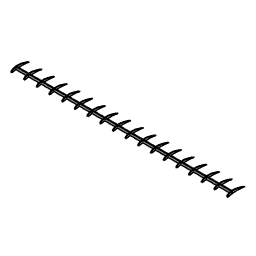
Boeing wing v1 (Autodesk Fusion 360 design; units mm, degrees)
Autodesk Fusion 360 part; units mm, degrees
note: some values were not read from the file. Set by a fixed rule: which sketch regions a step uses.
sketch "E423_1.0" plane through (0, 0, 0) normal (1, 0, 0) x (0, 0, -1)
  spline S0 degree 5 poles (0, 100) (-0.0021, 100.0005) (-0.0141, 99.9805) (-0.0559, 99.8873) (-0.1498, 99.6703) (-0.2899, 99.3695) (-0.4368, 99.0842) (-0.5908, 98.8088) (-0.7588, 98.5154) (-0.9439, 98.1889) (-1.1433, 97.8316) (-1.352, 97.4534) (-1.5644, 97.0669) (-1.7766, 96.6789) (-1.9869, 96.2896) (-2.1952, 95.8959) (-2.4017, 95.4928) (-2.607, 95.0764) (-2.8112, 94.6453) (-3.0137, 94.2001) (-3.2143, 93.7424) (-3.4125, 93.2744) (-3.6081, 92.7977) (-3.8013, 92.3132) (-3.9926, 91.8213) (-4.1824, 91.3216) (-4.3714, 90.8138) (-4.5601, 90.2978) (-4.7489, 89.7736) (-4.9377, 89.2414) (-5.1267, 88.7019) (-5.3157, 88.1556) (-5.5046, 87.6032) (-5.6933, 87.0452) (-5.8819, 86.4818) (-6.0702, 85.9134) (-6.2583, 85.34) (-6.4462, 84.7617) (-6.634, 84.1786) (-6.8217, 83.5907) (-7.0093, 82.9982) (-7.1967, 82.4013) (-7.3839, 81.8002) (-7.5709, 81.1951) (-7.7576, 80.5861) (-7.9439, 79.9736) (-8.1298, 79.3577) (-8.3152, 78.7385) (-8.5002, 78.1162) (-8.6845, 77.4909) (-8.8682, 76.8626) (-9.0513, 76.2315) (-9.2336, 75.5977) (-9.4152, 74.9612) (-9.596, 74.3223) (-9.7758, 73.681) (-9.9548, 73.0374) (-10.1328, 72.3916) (-10.3098, 71.7438) (-10.4856, 71.0941) (-10.6604, 70.4425) (-10.8339, 69.7892) (-11.0061, 69.1343) (-11.177, 68.4777) (-11.3465, 67.8197) (-11.5145, 67.1603) (-11.6809, 66.4996) (-11.8456, 65.8377) (-12.0086, 65.1746) (-12.1697, 64.5105) (-12.3289, 63.8455) (-12.4861, 63.1796) (-12.6411, 62.513) (-12.794, 61.8456) (-12.9446, 61.1777) (-13.0928, 60.5092) (-13.2386, 59.8402) (-13.3819, 59.1708) (-13.5226, 58.5011) (-13.6606, 57.8311) (-13.7958, 57.1609) (-13.9281, 56.4907) (-14.0573, 55.8205) (-14.1834, 55.1503) (-14.3061, 54.4803) (-14.4254, 53.8106) (-14.5409, 53.1412) (-14.6526, 52.4721) (-14.7601, 51.8034) (-14.8634, 51.1351) (-14.9621, 50.4673) (-15.0562, 49.7999) (-15.1453, 49.133) (-15.2294, 48.4665) (-15.3085, 47.8005) (-15.3823, 47.135) (-15.4509, 46.4699) (-15.5142, 45.8053) (-15.5722, 45.1412) (-15.6248, 44.4777) (-15.6722, 43.8147) (-15.7141, 43.1524) (-15.7507, 42.4907) (-15.7819, 41.8299) (-15.8077, 41.1698) (-15.8281, 40.5107) (-15.8431, 39.8526) (-15.8526, 39.1955) (-15.8567, 38.5395) (-15.8553, 37.8847) (-15.8485, 37.2311) (-15.8364, 36.5788) (-15.8188, 35.9278) (-15.7958, 35.2782) (-15.7674, 34.6301) (-15.7337, 33.9835) (-15.6946, 33.3387) (-15.6501, 32.6956) (-15.6003, 32.0543) (-15.5451, 31.4149) (-15.4846, 30.7776) (-15.4187, 30.1423) (-15.3476, 29.5091) (-15.2711, 28.8782) (-15.1893, 28.2495) (-15.1023, 27.6231) (-15.0101, 26.9992) (-14.9128, 26.3778) (-14.8103, 25.759) (-14.7029, 25.143) (-14.5905, 24.5298) (-14.4731, 23.9196) (-14.351, 23.3125) (-14.224, 22.7085) (-14.0923, 22.1078) (-13.9558, 21.5106) (-13.8146, 20.9168) (-13.6687, 20.3268) (-13.5181, 19.7405) (-13.3628, 19.1581) (-13.2028, 18.5797) (-13.0381, 18.0056) (-12.8687, 17.4357) (-12.6946, 16.8704) (-12.5159, 16.3097) (-12.3324, 15.7538) (-12.1444, 15.2029) (-11.9517, 14.6571) (-11.7543, 14.1166) (-11.5524, 13.5816) (-11.3459, 13.0522) (-11.1347, 12.5286) (-10.9189, 12.0109) (-10.6985, 11.4994) (-10.4735, 10.9943) (-10.2439, 10.4956) (-10.0096, 10.0037) (-9.7708, 9.5188) (-9.5273, 9.0412) (-9.2793, 8.571) (-9.0267, 8.1087) (-8.7697, 7.6544) (-8.5081, 7.2084) (-8.242, 6.771) (-7.9714, 6.3424) (-7.6963, 5.9229) (-7.4168, 5.513) (-7.1328, 5.1129) (-6.8444, 4.7231) (-6.5517, 4.3441) (-6.2547, 3.9762) (-5.9535, 3.62) (-5.6482, 3.2758) (-5.339, 2.9439) (-5.026, 2.625) (-4.7093, 2.3195) (-4.3891, 2.0282) (-4.0654, 1.7521) (-3.7383, 1.4922) (-3.4081, 1.2494) (-3.0753, 1.0245) (-2.7405, 0.8182) (-2.4045, 0.631) (-2.068, 0.4639) (-1.731, 0.3184) (-1.3931, 0.1973) (-1.0564, 0.103) (-0.7276, 0.0376) (-0.4228, 0.002) (-0.1632, -0.0059) (0.0354, 0.0078) (0.1775, 0.0302) (0.2843, 0.0476) (0.4091, 0.0826) (0.5351, 0.1305) (0.5811, 0.1515) (0.6519, 0.1886) (0.7136, 0.2323) (0.761, 0.2722) (0.8195, 0.3458) (0.8528, 0.3794) (0.9164, 0.4784) (0.9928, 0.6103) (1.0394, 0.7024) (1.101, 0.8594) (1.1715, 1.0486) (1.2233, 1.1907) (1.263, 1.3363) (1.3115, 1.5827) (1.3717, 1.9493) (1.4357, 2.4065) (1.4906, 2.9015) (1.5254, 3.3859) (1.537, 3.8426) (1.5274, 4.2759) (1.5021, 4.7023) (1.4672, 5.142) (1.427, 5.6084) (1.3827, 6.1039) (1.334, 6.6247) (1.2793, 7.163) (1.2169, 7.7103) (1.1456, 8.2603) (1.0652, 8.8106) (0.9763, 9.362) (0.8798, 9.9165) (0.7769, 10.4775) (0.6688, 11.0479) (0.5564, 11.6293) (0.44, 12.2223) (0.3199, 12.8262) (0.1963, 13.44) (0.0692, 14.0622) (-0.0614, 14.6916) (-0.1951, 15.3272) (-0.3316, 15.9686) (-0.4704, 16.6157) (-0.6109, 17.2689) (-0.7524, 17.9285) (-0.8944, 18.595) (-1.0364, 19.2686) (-1.178, 19.9494) (-1.3187, 20.6373) (-1.4584, 21.3321) (-1.5969, 22.0334) (-1.734, 22.7408) (-1.8696, 23.4538) (-2.0037, 24.1721) (-2.1361, 24.8953) (-2.2667, 25.6233) (-2.3954, 26.356) (-2.5219, 27.0932) (-2.6461, 27.8348) (-2.768, 28.581) (-2.8871, 29.3315) (-3.0035, 30.0864) (-3.1169, 30.8455) (-3.2271, 31.6086) (-3.334, 32.3756) (-3.4373, 33.1464) (-3.537, 33.9205) (-3.6328, 34.6979) (-3.7247, 35.4783) (-3.8125, 36.2614) (-3.8962, 37.047) (-3.9757, 37.8349) (-4.0509, 38.6249) (-4.1218, 39.4168) (-4.1886, 40.2103) (-4.251, 41.0052) (-4.3093, 41.8014) (-4.3636, 42.5986) (-4.4138, 43.3968) (-4.4601, 44.1956) (-4.5027, 44.9951) (-4.5417, 45.7949) (-4.5772, 46.595) (-4.6094, 47.3953) (-4.6383, 48.1955) (-4.6641, 48.9956) (-4.6868, 49.7956) (-4.7066, 50.5952) (-4.7235, 51.3944) (-4.7375, 52.1931) (-4.7486, 52.9912) (-4.757, 53.7886) (-4.7625, 54.5852) (-4.7653, 55.381) (-4.7653, 56.1759) (-4.7626, 56.9698) (-4.7572, 57.7626) (-4.749, 58.5542) (-4.7381, 59.3445) (-4.7246, 60.1334) (-4.7083, 60.9208) (-4.6893, 61.7067) (-4.6675, 62.4907) (-4.643, 63.273) (-4.6157, 64.0532) (-4.5856, 64.8313) (-4.5526, 65.6072) (-4.5169, 66.3806) (-4.4783, 67.1516) (-4.4368, 67.9198) (-4.3925, 68.6853) (-4.3454, 69.4479) (-4.2956, 70.2074) (-4.2429, 70.9637) (-4.1876, 71.7167) (-4.1296, 72.4662) (-4.0691, 73.2121) (-4.0062, 73.9541) (-3.9408, 74.692) (-3.8733, 75.4257) (-3.8036, 76.155) (-3.7319, 76.8796) (-3.6583, 77.5994) (-3.5828, 78.3144) (-3.5056, 79.0244) (-3.4265, 79.7294) (-3.3458, 80.4295) (-3.2633, 81.1245) (-3.1792, 81.8143) (-3.0936, 82.4989) (-3.0064, 83.178) (-2.9178, 83.8512) (-2.828, 84.5182) (-2.7372, 85.1783) (-2.6455, 85.8312) (-2.5531, 86.4765) (-2.46, 87.1139) (-2.3662, 87.7434) (-2.2717, 88.3655) (-2.1762, 88.9803) (-2.0795, 89.5885) (-1.9817, 90.1902) (-1.8828, 90.7851) (-1.783, 91.3726) (-1.683, 91.9512) (-1.5834, 92.519) (-1.485, 93.0737) (-1.3883, 93.6141) (-1.2935, 94.1394) (-1.2, 94.6507) (-1.1064, 95.1508) (-1.0112, 95.6433) (-0.9131, 96.1306) (-0.8119, 96.6128) (-0.709, 97.0855) (-0.6082, 97.5386) (-0.5141, 97.9598) (-0.4296, 98.3413) (-0.3539, 98.6832) (-0.2795, 99.003) (-0.1955, 99.3254) (-0.1004, 99.6525) (-0.0298, 99.88) (-0.0015, 99.9772) (0.0021, 99.9995) (0, 100) knots 0 0 0 0 0 0 0.0028169 0.0056338 0.0084507 0.01126761 0.01408451 0.01690141 0.01971831 0.02253521 0.02535211 0.02816901 0.03098592 0.03380282 0.03661972 0.03943662 0.04225352 0.04507042 0.04788732 0.05070423 0.05352113 0.05633803 0.05915493 0.06197183 0.06478873 0.06760563 0.07042254 0.07323944 0.07605634 0.07887324 0.08169014 0.08450704 0.08732394 0.09014085 0.09295775 0.09577465 0.09859155 0.10140845 0.10422535 0.10704225 0.10985915 0.11267606 0.11549296 0.11830986 0.12112676 0.12394366 0.12676056 0.12957746 0.13239437 0.13521127 0.13802817 0.14084507 0.14366197 0.14647887 0.14929577 0.15211268 0.15492958 0.15774648 0.16056338 0.16338028 0.16619718 0.16901408 0.17183099 0.17464789 0.17746479 0.18028169 0.18309859 0.18591549 0.18873239 0.1915493 0.1943662 0.1971831 0.2 0.2028169 0.2056338 0.2084507 0.21126761 0.21408451 0.21690141 0.21971831 0.22253521 0.22535211 0.22816901 0.23098592 0.23380282 0.23661972 0.23943662 0.24225352 0.24507042 0.24788732 0.25070423 0.25352113 0.25633803 0.25915493 0.26197183 0.26478873 0.26760563 0.27042254 0.27323944 0.27605634 0.27887324 0.28169014 0.28450704 0.28732394 0.29014085 0.29295775 0.29577465 0.29859155 0.30140845 0.30422535 0.30704225 0.30985915 0.31267606 0.31549296 0.31830986 0.32112676 0.32394366 0.32676056 0.32957746 0.33239437 0.33521127 0.33802817 0.34084507 0.34366197 0.34647887 0.34929577 0.35211268 0.35492958 0.35774648 0.36056338 0.36338028 0.36619718 0.36901408 0.37183099 0.37464789 0.37746479 0.38028169 0.38309859 0.38591549 0.38873239 0.3915493 0.3943662 0.3971831 0.4 0.4028169 0.4056338 0.4084507 0.41126761 0.41408451 0.41690141 0.41971831 0.42253521 0.42535211 0.42816901 0.43098592 0.43380282 0.43661972 0.43943662 0.44225352 0.44507042 0.44788732 0.45070423 0.45352113 0.45633803 0.45915493 0.46197183 0.46478873 0.46760563 0.47042254 0.47323944 0.47605634 0.47887324 0.48169014 0.48450704 0.48732394 0.49014085 0.49295775 0.49577465 0.49859155 0.50140845 0.50422535 0.50704225 0.50985915 0.51267606 0.51549296 0.51830986 0.52112676 0.52394366 0.52676056 0.52957746 0.53239437 0.53521127 0.53802817 0.54084507 0.54366197 0.54647887 0.54929577 0.55211268 0.55492958 0.55774648 0.56056338 0.56338028 0.56619718 0.56901408 0.57183099 0.57464789 0.57746479 0.58028169 0.58309859 0.58591549 0.58873239 0.5915493 0.5943662 0.5971831 0.6 0.6028169 0.6056338 0.6084507 0.61126761 0.61408451 0.61690141 0.61971831 0.62253521 0.62535211 0.62816901 0.63098592 0.63380282 0.63661972 0.63943662 0.64225352 0.64507042 0.64788732 0.65070423 0.65352113 0.65633803 0.65915493 0.66197183 0.66478873 0.66760563 0.67042254 0.67323944 0.67605634 0.67887324 0.68169014 0.68450704 0.68732394 0.69014085 0.69295775 0.69577465 0.69859155 0.70140845 0.70422535 0.70704225 0.70985915 0.71267606 0.71549296 0.71830986 0.72112676 0.72394366 0.72676056 0.72957746 0.73239437 0.73521127 0.73802817 0.74084507 0.74366197 0.74647887 0.74929577 0.75211268 0.75492958 0.75774648 0.76056338 0.76338028 0.76619718 0.76901408 0.77183099 0.77464789 0.77746479 0.78028169 0.78309859 0.78591549 0.78873239 0.7915493 0.7943662 0.7971831 0.8 0.8028169 0.8056338 0.8084507 0.81126761 0.81408451 0.81690141 0.81971831 0.82253521 0.82535211 0.82816901 0.83098592 0.83380282 0.83661972 0.83943662 0.84225352 0.84507042 0.84788732 0.85070423 0.85352113 0.85633803 0.85915493 0.86197183 0.86478873 0.86760563 0.87042254 0.87323944 0.87605634 0.87887324 0.88169014 0.88450704 0.88732394 0.89014085 0.89295775 0.89577465 0.89859155 0.90140845 0.90422535 0.90704225 0.90985915 0.91267606 0.91549296 0.91830986 0.92112676 0.92394366 0.92676056 0.92957746 0.93239437 0.93521127 0.93802817 0.94084507 0.94366197 0.94647887 0.94929577 0.95211268 0.95492958 0.95774648 0.96056338 0.96338028 0.96619718 0.96901408 0.97183099 0.97464789 0.97746479 0.98028169 0.98309859 0.98591549 0.98873239 0.9915493 0.9943662 0.9971831 1 1 1 1 1 1
  point P0 (-0.159, 99.655)
  point P1 (-0.65, 98.706)
  point P2 (-1.434, 97.304)
  point P3 (-2.381, 95.53)
  point P4 (-3.376, 93.358)
  point P5 (-4.4, 90.734)
  point P6 (-5.481, 87.671)
  point P7 (-6.62, 84.221)
  point P8 (-7.803, 80.436)
  point P9 (-9.01, 76.373)
  point P10 (-10.215, 72.09)
  point P11 (-11.391, 67.644)
  point P12 (-12.506, 63.092)
  point P13 (-13.524, 58.491)
  point P14 (-14.41, 53.893)
  point P15 (-15.116, 49.347)
  point P16 (-15.593, 44.87)
  point P17 (-15.828, 40.464)
  point P18 (-15.824, 36.149)
  point P19 (-15.59, 31.947)
  point P20 (-15.138, 27.885)
  point P21 (-14.485, 23.987)
  point P22 (-13.657, 20.286)
  point P23 (-12.676, 16.816)
  point P24 (-11.562, 13.611)
  point P25 (-10.337, 10.7)
  point P26 (-9.023, 8.106)
  point P27 (-7.646, 5.852)
  point P28 (-6.232, 3.953)
  point P29 (-4.812, 2.421)
  point P30 (-3.419, 1.262)
  point P31 (-2.093, 0.481)
  point P32 (-0.879, 0.071)
  point P33 (-0.088, 0.002)
  point P34 (0.192, 0.033)
  point P35 (0.362, 0.071)
  point P36 (0.518, 0.125)
  point P37 (0.59, 0.157)
  point P38 (0.656, 0.194)
  point P39 (0.717, 0.237)
  point P40 (0.771, 0.288)
  point P41 (0.823, 0.348)
  point P42 (0.874, 0.415)
  point P43 (0.969, 0.571)
  point P44 (1.057, 0.751)
  point P45 (1.177, 1.065)
  point P46 (1.266, 1.365)
  point P47 (1.485, 2.892)
  point P48 (1.482, 4.947)
  point P49 (1.236, 7.533)
  point P50 (0.74, 10.67)
  point P51 (0.002, 14.385)
  point P52 (-0.922, 18.727)
  point P53 (-1.913, 23.688)
  point P54 (-2.865, 29.196)
  point P55 (-3.687, 35.163)
  point P56 (-4.283, 41.449)
  point P57 (-4.626, 47.867)
  point P58 (-4.76, 54.275)
  point P59 (-4.715, 60.579)
  point P60 (-4.501, 66.69)
  point P61 (-4.126, 72.503)
  point P62 (-3.625, 77.912)
  point P63 (-3.05, 82.836)
  point P64 (-2.444, 87.219)
  point P65 (-1.844, 91.012)
  point P66 (-1.286, 94.179)
  point P67 (-0.794, 96.692)
  point P68 (-0.39, 98.519)
  point P69 (-0.106, 99.629)
extrude "Extrude1" add sketch "E423_1.0" along normal blind 3 makes body 1
sketch "Sketch2" plane through (3, 0, 0) normal (1, 0, 0) x (0, 1, 0)
  spline S0 degree 5 poles (100, 0) (100.0005, 0.0021) (99.9805, 0.0141) (99.8873, 0.0559) (99.6703, 0.1498) (99.3695, 0.2899) (99.0842, 0.4368) (98.8088, 0.5908) (98.5154, 0.7588) (98.1889, 0.9439) (97.8316, 1.1433) (97.4534, 1.352) (97.0669, 1.5644) (96.6789, 1.7766) (96.2896, 1.9869) (95.8959, 2.1952) (95.4928, 2.4017) (95.0764, 2.607) (94.6453, 2.8112) (94.2001, 3.0137) (93.7424, 3.2143) (93.2744, 3.4125) (92.7977, 3.6081) (92.3132, 3.8013) (91.8213, 3.9926) (91.3216, 4.1824) (90.8138, 4.3714) (90.2978, 4.5601) (89.7736, 4.7489) (89.2414, 4.9377) (88.7019, 5.1267) (88.1556, 5.3157) (87.6032, 5.5046) (87.0452, 5.6933) (86.4818, 5.8819) (85.9134, 6.0702) (85.34, 6.2583) (84.7617, 6.4462) (84.1786, 6.634) (83.5907, 6.8217) (82.9982, 7.0093) (82.4013, 7.1967) (81.8002, 7.3839) (81.1951, 7.5709) (80.5861, 7.7576) (79.9736, 7.9439) (79.3577, 8.1298) (78.7385, 8.3152) (78.1162, 8.5002) (77.4909, 8.6845) (76.8626, 8.8682) (76.2315, 9.0513) (75.5977, 9.2336) (74.9612, 9.4152) (74.3223, 9.596) (73.681, 9.7758) (73.0374, 9.9548) (72.3916, 10.1328) (71.7438, 10.3098) (71.0941, 10.4856) (70.4425, 10.6604) (69.7892, 10.8339) (69.1343, 11.0061) (68.4777, 11.177) (67.8197, 11.3465) (67.1603, 11.5145) (66.4996, 11.6809) (65.8377, 11.8456) (65.1746, 12.0086) (64.5105, 12.1697) (63.8455, 12.3289) (63.1796, 12.4861) (62.513, 12.6411) (61.8456, 12.794) (61.1777, 12.9446) (60.5092, 13.0928) (59.8402, 13.2386) (59.1708, 13.3819) (58.5011, 13.5226) (57.8311, 13.6606) (57.1609, 13.7958) (56.4907, 13.9281) (55.8205, 14.0573) (55.1503, 14.1834) (54.4803, 14.3061) (53.8106, 14.4254) (53.1412, 14.5409) (52.4721, 14.6526) (51.8034, 14.7601) (51.1351, 14.8634) (50.4673, 14.9621) (49.7999, 15.0562) (49.133, 15.1453) (48.4665, 15.2294) (47.8005, 15.3085) (47.135, 15.3823) (46.4699, 15.4509) (45.8053, 15.5142) (45.1412, 15.5722) (44.4777, 15.6248) (43.8147, 15.6722) (43.1524, 15.7141) (42.4907, 15.7507) (41.8299, 15.7819) (41.1698, 15.8077) (40.5107, 15.8281) (39.8526, 15.8431) (39.1955, 15.8526) (38.5395, 15.8567) (37.8847, 15.8553) (37.2311, 15.8485) (36.5788, 15.8364) (35.9278, 15.8188) (35.2782, 15.7958) (34.6301, 15.7674) (33.9835, 15.7337) (33.3387, 15.6946) (32.6956, 15.6501) (32.0543, 15.6003) (31.4149, 15.5451) (30.7776, 15.4846) (30.1423, 15.4187) (29.5091, 15.3476) (28.8782, 15.2711) (28.2495, 15.1893) (27.6231, 15.1023) (26.9992, 15.0101) (26.3778, 14.9128) (25.759, 14.8103) (25.143, 14.7029) (24.5298, 14.5905) (23.9196, 14.4731) (23.3125, 14.351) (22.7085, 14.224) (22.1078, 14.0923) (21.5106, 13.9558) (20.9168, 13.8146) (20.3268, 13.6687) (19.7405, 13.5181) (19.1581, 13.3628) (18.5797, 13.2028) (18.0056, 13.0381) (17.4357, 12.8687) (16.8704, 12.6946) (16.3097, 12.5159) (15.7538, 12.3324) (15.2029, 12.1444) (14.6571, 11.9517) (14.1166, 11.7543) (13.5816, 11.5524) (13.0522, 11.3459) (12.5286, 11.1347) (12.0109, 10.9189) (11.4994, 10.6985) (10.9943, 10.4735) (10.4956, 10.2439) (10.0037, 10.0096) (9.5188, 9.7708) (9.0412, 9.5273) (8.571, 9.2793) (8.1087, 9.0267) (7.6544, 8.7697) (7.2084, 8.5081) (6.771, 8.242) (6.3424, 7.9714) (5.9229, 7.6963) (5.513, 7.4168) (5.1129, 7.1328) (4.7231, 6.8444) (4.3441, 6.5517) (3.9762, 6.2547) (3.62, 5.9535) (3.2758, 5.6482) (2.9439, 5.339) (2.625, 5.026) (2.3195, 4.7093) (2.0282, 4.3891) (1.7521, 4.0654) (1.4922, 3.7383) (1.2494, 3.4081) (1.0245, 3.0753) (0.8182, 2.7405) (0.631, 2.4045) (0.4639, 2.068) (0.3184, 1.731) (0.1973, 1.3931) (0.103, 1.0564) (0.0376, 0.7276) (0.002, 0.4228) (-0.0059, 0.1632) (0.0078, -0.0354) (0.0302, -0.1775) (0.0476, -0.2843) (0.0826, -0.4091) (0.1305, -0.5351) (0.1515, -0.5811) (0.1886, -0.6519) (0.2323, -0.7136) (0.2722, -0.761) (0.3458, -0.8195) (0.3794, -0.8528) (0.4784, -0.9164) (0.6103, -0.9928) (0.7024, -1.0394) (0.8594, -1.101) (1.0486, -1.1715) (1.1907, -1.2233) (1.3363, -1.263) (1.5827, -1.3115) (1.9493, -1.3717) (2.4065, -1.4357) (2.9015, -1.4906) (3.3859, -1.5254) (3.8426, -1.537) (4.2759, -1.5274) (4.7023, -1.5021) (5.142, -1.4672) (5.6084, -1.427) (6.1039, -1.3827) (6.6247, -1.334) (7.163, -1.2793) (7.7103, -1.2169) (8.2603, -1.1456) (8.8106, -1.0652) (9.362, -0.9763) (9.9165, -0.8798) (10.4775, -0.7769) (11.0479, -0.6688) (11.6293, -0.5564) (12.2223, -0.44) (12.8262, -0.3199) (13.44, -0.1963) (14.0622, -0.0692) (14.6916, 0.0614) (15.3272, 0.1951) (15.9686, 0.3316) (16.6157, 0.4704) (17.2689, 0.6109) (17.9285, 0.7524) (18.595, 0.8944) (19.2686, 1.0364) (19.9494, 1.178) (20.6373, 1.3187) (21.3321, 1.4584) (22.0334, 1.5969) (22.7408, 1.734) (23.4538, 1.8696) (24.1721, 2.0037) (24.8953, 2.1361) (25.6233, 2.2667) (26.356, 2.3954) (27.0932, 2.5219) (27.8348, 2.6461) (28.581, 2.768) (29.3315, 2.8871) (30.0864, 3.0035) (30.8455, 3.1169) (31.6086, 3.2271) (32.3756, 3.334) (33.1464, 3.4373) (33.9205, 3.537) (34.6979, 3.6328) (35.4783, 3.7247) (36.2614, 3.8125) (37.047, 3.8962) (37.8349, 3.9757) (38.6249, 4.0509) (39.4168, 4.1218) (40.2103, 4.1886) (41.0052, 4.251) (41.8014, 4.3093) (42.5986, 4.3636) (43.3968, 4.4138) (44.1956, 4.4601) (44.9951, 4.5027) (45.7949, 4.5417) (46.595, 4.5772) (47.3953, 4.6094) (48.1955, 4.6383) (48.9956, 4.6641) (49.7956, 4.6868) (50.5952, 4.7066) (51.3944, 4.7235) (52.1931, 4.7375) (52.9912, 4.7486) (53.7886, 4.757) (54.5852, 4.7625) (55.381, 4.7653) (56.1759, 4.7653) (56.9698, 4.7626) (57.7626, 4.7572) (58.5542, 4.749) (59.3445, 4.7381) (60.1334, 4.7246) (60.9208, 4.7083) (61.7067, 4.6893) (62.4907, 4.6675) (63.273, 4.643) (64.0532, 4.6157) (64.8313, 4.5856) (65.6072, 4.5526) (66.3806, 4.5169) (67.1516, 4.4783) (67.9198, 4.4368) (68.6853, 4.3925) (69.4479, 4.3454) (70.2074, 4.2956) (70.9637, 4.2429) (71.7167, 4.1876) (72.4662, 4.1296) (73.2121, 4.0691) (73.9541, 4.0062) (74.692, 3.9408) (75.4257, 3.8733) (76.155, 3.8036) (76.8796, 3.7319) (77.5994, 3.6583) (78.3144, 3.5828) (79.0244, 3.5056) (79.7294, 3.4265) (80.4295, 3.3458) (81.1245, 3.2633) (81.8143, 3.1792) (82.4989, 3.0936) (83.178, 3.0064) (83.8512, 2.9178) (84.5182, 2.828) (85.1783, 2.7372) (85.8312, 2.6455) (86.4765, 2.5531) (87.1139, 2.46) (87.7434, 2.3662) (88.3655, 2.2717) (88.9803, 2.1762) (89.5885, 2.0795) (90.1902, 1.9817) (90.7851, 1.8828) (91.3726, 1.783) (91.9512, 1.683) (92.519, 1.5834) (93.0737, 1.485) (93.6141, 1.3883) (94.1394, 1.2935) (94.6507, 1.2) (95.1508, 1.1064) (95.6433, 1.0112) (96.1306, 0.9131) (96.6128, 0.8119) (97.0855, 0.709) (97.5386, 0.6082) (97.9598, 0.5141) (98.3413, 0.4296) (98.6832, 0.3539) (99.003, 0.2795) (99.3254, 0.1955) (99.6525, 0.1004) (99.88, 0.0298) (99.9772, 0.0015) (99.9995, -0.0021) (100, 0) knots 0 0 0 0 0 0 0.0028169 0.0056338 0.0084507 0.01126761 0.01408451 0.01690141 0.01971831 0.02253521 0.02535211 0.02816901 0.03098592 0.03380282 0.03661972 0.03943662 0.04225352 0.04507042 0.04788732 0.05070423 0.05352113 0.05633803 0.05915493 0.06197183 0.06478873 0.06760563 0.07042254 0.07323944 0.07605634 0.07887324 0.08169014 0.08450704 0.08732394 0.09014085 0.09295775 0.09577465 0.09859155 0.10140845 0.10422535 0.10704225 0.10985915 0.11267606 0.11549296 0.11830986 0.12112676 0.12394366 0.12676056 0.12957746 0.13239437 0.13521127 0.13802817 0.14084507 0.14366197 0.14647887 0.14929577 0.15211268 0.15492958 0.15774648 0.16056338 0.16338028 0.16619718 0.16901408 0.17183099 0.17464789 0.17746479 0.18028169 0.18309859 0.18591549 0.18873239 0.1915493 0.1943662 0.1971831 0.2 0.2028169 0.2056338 0.2084507 0.21126761 0.21408451 0.21690141 0.21971831 0.22253521 0.22535211 0.22816901 0.23098592 0.23380282 0.23661972 0.23943662 0.24225352 0.24507042 0.24788732 0.25070423 0.25352113 0.25633803 0.25915493 0.26197183 0.26478873 0.26760563 0.27042254 0.27323944 0.27605634 0.27887324 0.28169014 0.28450704 0.28732394 0.29014085 0.29295775 0.29577465 0.29859155 0.30140845 0.30422535 0.30704225 0.30985915 0.31267606 0.31549296 0.31830986 0.32112676 0.32394366 0.32676056 0.32957746 0.33239437 0.33521127 0.33802817 0.34084507 0.34366197 0.34647887 0.34929577 0.35211268 0.35492958 0.35774648 0.36056338 0.36338028 0.36619718 0.36901408 0.37183099 0.37464789 0.37746479 0.38028169 0.38309859 0.38591549 0.38873239 0.3915493 0.3943662 0.3971831 0.4 0.4028169 0.4056338 0.4084507 0.41126761 0.41408451 0.41690141 0.41971831 0.42253521 0.42535211 0.42816901 0.43098592 0.43380282 0.43661972 0.43943662 0.44225352 0.44507042 0.44788732 0.45070423 0.45352113 0.45633803 0.45915493 0.46197183 0.46478873 0.46760563 0.47042254 0.47323944 0.47605634 0.47887324 0.48169014 0.48450704 0.48732394 0.49014085 0.49295775 0.49577465 0.49859155 0.50140845 0.50422535 0.50704225 0.50985915 0.51267606 0.51549296 0.51830986 0.52112676 0.52394366 0.52676056 0.52957746 0.53239437 0.53521127 0.53802817 0.54084507 0.54366197 0.54647887 0.54929577 0.55211268 0.55492958 0.55774648 0.56056338 0.56338028 0.56619718 0.56901408 0.57183099 0.57464789 0.57746479 0.58028169 0.58309859 0.58591549 0.58873239 0.5915493 0.5943662 0.5971831 0.6 0.6028169 0.6056338 0.6084507 0.61126761 0.61408451 0.61690141 0.61971831 0.62253521 0.62535211 0.62816901 0.63098592 0.63380282 0.63661972 0.63943662 0.64225352 0.64507042 0.64788732 0.65070423 0.65352113 0.65633803 0.65915493 0.66197183 0.66478873 0.66760563 0.67042254 0.67323944 0.67605634 0.67887324 0.68169014 0.68450704 0.68732394 0.69014085 0.69295775 0.69577465 0.69859155 0.70140845 0.70422535 0.70704225 0.70985915 0.71267606 0.71549296 0.71830986 0.72112676 0.72394366 0.72676056 0.72957746 0.73239437 0.73521127 0.73802817 0.74084507 0.74366197 0.74647887 0.74929577 0.75211268 0.75492958 0.75774648 0.76056338 0.76338028 0.76619718 0.76901408 0.77183099 0.77464789 0.77746479 0.78028169 0.78309859 0.78591549 0.78873239 0.7915493 0.7943662 0.7971831 0.8 0.8028169 0.8056338 0.8084507 0.81126761 0.81408451 0.81690141 0.81971831 0.82253521 0.82535211 0.82816901 0.83098592 0.83380282 0.83661972 0.83943662 0.84225352 0.84507042 0.84788732 0.85070423 0.85352113 0.85633803 0.85915493 0.86197183 0.86478873 0.86760563 0.87042254 0.87323944 0.87605634 0.87887324 0.88169014 0.88450704 0.88732394 0.89014085 0.89295775 0.89577465 0.89859155 0.90140845 0.90422535 0.90704225 0.90985915 0.91267606 0.91549296 0.91830986 0.92112676 0.92394366 0.92676056 0.92957746 0.93239437 0.93521127 0.93802817 0.94084507 0.94366197 0.94647887 0.94929577 0.95211268 0.95492958 0.95774648 0.96056338 0.96338028 0.96619718 0.96901408 0.97183099 0.97464789 0.97746479 0.98028169 0.98309859 0.98591549 0.98873239 0.9915493 0.9943662 0.9971831 1 1 1 1 1 1
  line L0 (0, 15) -> (26, 15)
  line L1 (25, 20) -> (29, 20)
  line L2 (29, 20) -> (29, 8)
  line L3 (29, 8) -> (25, 8)
  line L4 (25, 8) -> (25, 20)
  constraint horizontal L0
  constraint horizontal L1
  constraint vertical L2
  constraint horizontal L3
  constraint vertical L4
extrude "Extrude2" cut sketch "Sketch2" against normal blind 3 contours S0 L2 L3 L4 picked at (27.6667, 12.6536) bodies 1
pattern_linear "R-Pattern1" count 18 spacing 70.4118 along (1, 0, 0) of bodies 1 makes body 2 at (70.4118, 45.0195, 7.9914) makes body 3 at (140.8235, 45.0195, 7.9914) makes body 4 at (211.2353, 45.0195, 7.9914) makes body 5 at (281.6471, 45.0195, 7.9914) makes body 6 at (352.0588, 45.0195, 7.9914) makes body 7 at (422.4706, 45.0195, 7.9914) makes body 8 at (492.8824, 45.0195, 7.9914) makes body 9 at (563.2941, 45.0195, 7.9914) makes body 10 at (633.7059, 45.0195, 7.9914) makes body 11 at (704.1176, 45.0195, 7.9914) makes body 12 at (774.5294, 45.0195, 7.9914) makes body 13 at (844.9412, 45.0195, 7.9914) makes body 14 at (915.3529, 45.0195, 7.9914) makes body 15 at (985.7647, 45.0195, 7.9914) makes body 16 at (1056.1765, 45.0195, 7.9914) makes body 17 at (1126.5882, 45.0195, 7.9914) makes body 18 at (1197, 45.0195, 7.9914)
sketch "Sketch3" plane through (0, 0, 0) normal (1, 0, 0) x (0, 1, 0)
  line L0 (29, 15.285) -> (25, 15.285)
  line L1 (25, 15.285) -> (25, 2)
  line L2 (25, 2) -> (29, 2)
  line L3 (29, 2) -> (29, 15.285)
  constraint horizontal L0
  constraint vertical L1
  constraint horizontal L2
  constraint vertical L3
extrude "Extrude3" add sketch "Sketch3" along normal blind 1200 separate body makes body 19
